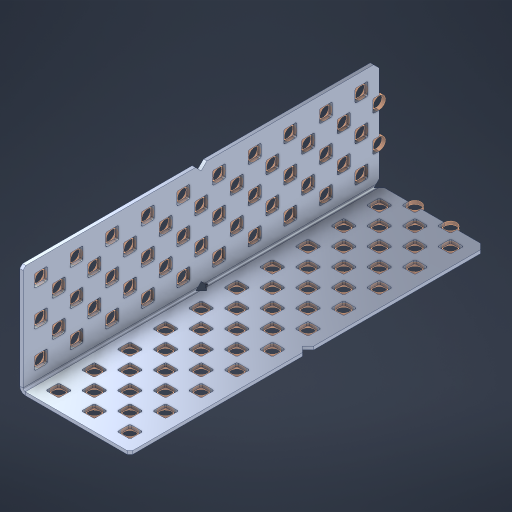
# Autodesk Inventor part: Alu C 1x2x1x35
Saved by Autodesk Inventor 2023 (Build 270158000, 158)
## iProperties
Created: 2022-07-28
Part Number: Alu C 1x2x1x35
Material: Generic
Document SubType Name: Sheet Metal
Designer: ylu12
Density: 1 g/cm^3
Sheet Metal Rule: Default
Appearance: Steel
Author: ylu12
Autodesk Inventor part; units mm, degrees
ref_plane "YZ Plane" through (0, 0, 0) normal (1, 0, 0) x (0, 1, 0)
ref_plane "XZ Plane" through (0, 0, 0) normal (0, 1, 0) x (-1, 0, 0)
sketch "Sketch1" plane through (0, 0, 0) normal (0, 1, 0) x (-1, 0, 0)
  line L0 (-19.05, 0) -> (19.05, 0)
  line L1 (19.05, 0) -> (19.05, -127)
  line L2 (19.05, -127) -> (-19.05, -127)
  line L3 (-19.05, -127) -> (-19.05, 0)
  line L4 (19.05, 0) -> (-19.05, -127) construction
  point P0 (0, 0)
  point P1 (0, 0)
  dimension "d0" = 38.1
  dimension "d1" = 127
  measures "d0" distance of L1.end L2.end
  measures "d1" distance of L0.end L1.end
extrude "Plate1" add sketch "Sketch1" along normal blind 1.1906
sketch "Sketch2" plane through (-19.05, 1.1906, 0) normal (-1, 0, 0) x (0, -1, 0)
  line L0 (0, -127) -> (0, 0)
  line L1 (0, 0) -> (-38.1, 0)
  line L2 (-38.1, 0) -> (-38.1, -127)
  line L3 (-38.1, -127) -> (0, -127)
  constraints: 6 end point, 1 horizontal, 1 perpendicular, 1 vertical
edge flange "Flanges" height 38.1 angle 90 thickness 1.1906 bend radius 0.7937 thickness toward (-1, 0, 0) relief tear relief width 1.1906 relief depth 0.5953 edges at (-19.05, 1.1906, -63.5) wall of the first edge with corners at (-19.05, 1.1906, -127) (-19.05, 1.1906, 0) (-19.05, 39.2906, 0) (-19.05, 39.2906, -127)
bend "Bend1"
corner "Corner1"
sketch "Sketch8" plane through (0, 0, 0) normal (0, -1, 0) x (1, 0, 0)
  line L0 (19.05, 0) -> (-18.2562, 0) construction
  line L1 (14.5034, -4.0386) -> (10.8966, -4.0386)
  line L2 (10.3886, -4.5466) -> (10.3886, -8.1534)
  line L3 (10.8966, -8.6614) -> (14.5034, -8.6614)
  line L4 (15.0114, -8.1534) -> (15.0114, -4.5466)
  arc A0 (15.0114, -4.5466) -> (14.5034, -4.0386) centre (14.5034, -4.5466) ccw
  arc A1 (14.5034, -8.6614) -> (15.0114, -8.1534) centre (14.5034, -8.1534) ccw
  arc A2 (10.3886, -8.1534) -> (10.8966, -8.6614) centre (10.8966, -8.1534) ccw
  arc A3 (10.8966, -4.0386) -> (10.3886, -4.5466) centre (10.8966, -4.5466) ccw
  line L5 (14.5034, -4.5466) -> (10.8966, -8.1534) construction
  line L6 (19.05, -127) -> (19.05, 0) construction
  point P0 (0, 0)
  point P1 (10.3886, -8.6614)
  point P2 (15.0114, -8.6614)
  point P3 (12.7, -6.35)
  dimension "d49" = 4.6228
  dimension "d50" = 0.508
  dimension "d52" = 6.35
  dimension "d131" = 6.35
  constraints: 10 end point, 8 point on circle, 8 tangent, 4 centre point, 4 point on line, 3 equal radius, 2 parallel, 2 perpendicular, 1 horizontal, 1 midpoint
  measures "d49" distance of point (15.011, -8.661) point (10.389, -8.661)
  measures "d50" radius of A0
  measures "d52" distance from line of L0 point (12.7, -6.35)
  measures "d131" distance from line of L6 point (12.7, -6.35)
extrude "Body Stamp" cut sketch "Sketch8" against normal blind 1.1906
sketch "Sketch9" plane through (0, 0, 0) normal (0, -1, 0) x (1, 0, 0)
  arc A0 (15.0114, -4.5466) -> (14.5034, -4.0386) centre (14.5034, -4.5466) ccw construction
  arc A1 (10.3886, -8.1534) -> (10.8966, -8.6614) centre (10.8966, -8.1534) ccw construction
  line L0 (14.5034, -4.5466) -> (10.8966, -8.1534) construction
  circle A2 centre (12.7, -6.35) radius 2.1844
  point P0 (0, 0)
  dimension "d55" = 4.3688
  constraints: 2 end point, 1 centre point, 1 midpoint
  measures "d55" diameter of A2
surface extrude "Body Circle" sketch "Sketch9" against normal up to surface (1.1906 mm away) shown yes curves A2
pattern_sketch "Body Pattern" of "Body Stamp", "Body Circle" from (12.7, 0, -6.35) copies at (0, 0, -6.35) at (-12.7, 0, -6.35) at (12.7, 0, -19.05) at (0, 0, -19.05) at (-12.7, 0, -19.05) at (12.7, 0, -31.75) at (0, 0, -31.75) at (-12.7, 0, -31.75) at (12.7, 0, -44.45) at (0, 0, -44.45) at (-12.7, 0, -44.45) at (12.7, 0, -57.15) at (0, 0, -57.15) at (-12.7, 0, -57.15) at (12.7, 0, -69.85) at (0, 0, -69.85) at (-12.7, 0, -69.85) at (12.7, 0, -82.55) at (0, 0, -82.55) at (-12.7, 0, -82.55) at (12.7, 0, -95.25) at (0, 0, -95.25) at (-12.7, 0, -95.25) at (12.7, 0, -107.95) at (0, 0, -107.95) at (-12.7, 0, -107.95) at (12.7, 0, -120.65) at (0, 0, -120.65) at (-12.7, 0, -120.65)
sketch "Sketch15" plane through (0, 0, 0) normal (0, -1, 0) x (1, 0, 0)
  line L0 (19.05, 0) -> (-18.2562, 0) construction
  line L1 (-4.5466, -10.3886) -> (-8.1534, -10.3886)
  line L2 (-8.6614, -10.8966) -> (-8.6614, -14.5034)
  line L3 (-8.1534, -15.0114) -> (-4.5466, -15.0114)
  line L4 (-4.0386, -14.5034) -> (-4.0386, -10.8966)
  arc A0 (-4.0386, -10.8966) -> (-4.5466, -10.3886) centre (-4.5466, -10.8966) ccw
  arc A1 (-4.5466, -15.0114) -> (-4.0386, -14.5034) centre (-4.5466, -14.5034) ccw
  arc A2 (-8.1534, -10.3886) -> (-8.6614, -10.8966) centre (-8.1534, -10.8966) ccw
  arc A3 (-8.6614, -14.5034) -> (-8.1534, -15.0114) centre (-8.1534, -14.5034) ccw
  line L5 (-4.5466, -10.8966) -> (-8.1534, -14.5034) construction
  line L6 (19.05, -127) -> (19.05, 0) construction
  point P0 (10.3187, 0)
  point P1 (0, 0)
  point P2 (-8.6614, -15.0114)
  point P3 (-4.0386, -15.0114)
  point P4 (-6.35, -12.7)
  dimension "d106" = 4.6228
  dimension "d107" = 0.508
  dimension "d140" = 12.7
  dimension "d141" = 25.4
  constraints: 10 end point, 8 point on circle, 8 tangent, 4 centre point, 4 point on line, 3 equal radius, 2 parallel, 2 perpendicular, 1 horizontal, 1 midpoint
  measures "d106" distance of point (-4.039, -15.011) point (-8.661, -15.011)
  measures "d107" radius of A0
  measures "d140" distance from line of L0 point (-6.35, -12.7)
  measures "d141" distance from line of L6 point (-6.35, -12.7)
extrude "Center Stamp" cut sketch "Sketch15" against normal blind 1.1906
sketch "Sketch16" plane through (0, 0, 0) normal (0, -1, 0) x (1, 0, 0)
  circle A0 centre (-6.35, -12.7) radius 2.1844
  arc A1 (-8.1534, -10.3886) -> (-8.6614, -10.8966) centre (-8.1534, -10.8966) ccw construction
  arc A2 (-4.0386, -10.8966) -> (-4.5466, -10.3886) centre (-4.5466, -10.8966) ccw construction
  line L0 (-4.5466, -10.8966) -> (-8.1534, -10.8966) construction
  arc A3 (-8.1534, -10.3886) -> (-8.6614, -10.8966) centre (-8.1534, -10.8966) ccw construction
  line L1 (-8.1534, -10.8966) -> (-6.35, -12.7) construction
  line L2 (-6.35, -12.7) -> (-4.5466, -10.8966) construction
  point P0 (0, 0)
  point P1 (10.3187, 0)
  dimension "d112" = 4.3688
  dimension "d145" = 1.8034
  constraints: 6 end point, 1 centre point, 1 horizontal, 1 perpendicular
  measures "d112" diameter of A0
  measures "d145" distance from line of L1.end L0
surface extrude "Center Circle" sketch "Sketch16" against normal up to surface (1.1906 mm away) shown yes curves A0
pattern_linear "Center Double" count 2 spacing 12.7 along (1, 0, 0) of "Center Stamp", "Center Circle"
pattern_linear "Center Pattern" count 10 spacing 12.7 along (0, 0, -1) of "Center Circle", "Center Stamp", "Center Double"
sketch "Arc Length" plane through (5.1594, 1.9844, 0) normal (0, 0, 1) x (1, 0, 0)
  line L0 (-25.4, 0) -> (-24.2094, 0) projected
  arc A0 (-25.4, 0) -> (-23.4156, -1.9844) centre (-23.4156, 0) ccw projected
  line L1 (-23.4156, -0.7938) -> (-23.4156, -1.9844) projected
  arc A1 (-24.2094, 0) -> (-23.4156, -0.7938) centre (-23.4156, 0) ccw projected
  point P0 (-5.1594, -1.9844)
  dimension "d126" = 1.2468
  dimension "d127" = 3.117
sketch "Sketch13" plane through (-20.2406, 26.5906, 317.5) normal (1, 0, 0) x (0, 0, -1)
  line L0 (378.968, 12.7) -> (381, 10.668)
  line L1 (381, 10.668) -> (383.032, 12.7)
  line L2 (378.968, 12.7) -> (383.032, 12.7)
  line L3 (381, -23.5903) -> (378.893, -25.6972)
  line L4 (378.893, -25.6972) -> (381, -27.8042)
  line L5 (381, -27.8042) -> (383.107, -25.6972)
  line L6 (383.107, -25.6972) -> (381, -23.5903)
  line L7 (381, -23.5903) -> (381, -27.8042) construction
  line L8 (381, 10.668) -> (381, -23.5903) construction
  line L9 (444.5, 12.7) -> (317.5, 12.7) projected
  line L10 (444.5, -24.6062) -> (317.5, -24.6062) construction
  line L11 (317.5, 12.7) -> (317.5, -24.6062) construction
  point P0 (444.5, -11.9062)
  point P1 (317.5, -26.5906)
  dimension "d86" = 4.2139
  dimension "d128" = 2.032
  dimension "d129" = 1.016
  dimension "d130" = 63.5
  constraints: 19 end point, 6 perpendicular, 2 vertical, 1 collinear, 1 other
  measures "d86" distance of L3.start L4.end
  measures "d128" distance from line of L2 L0.end
  measures "d130" distance between parallel lines of L11 L8
cut across bends "Notch" sketch "Sketch13" k factor 0.44
pattern_linear "Notch Pattern" count 2 spacing 63.5 along (0, 0, -1) of "Notch"
ref_plane "Diagonal Plane" through (-19.05, 1.1906, 0) normal (-0.7071068, 0.7071068, 0) x (0, 0, 1)
mirror "Everything Mirrored" about plane through (-19.05, 1.1906, 0) normal (-0.7071068, 0.7071068, 0) of "Body Stamp", "Body Circle", "Body Pattern", "Center Stamp", "Center Circle", "Center Pattern", "Notch", "Notch Pattern", "Center Double"
chamfer "End Chamfer" distance 1.016 angle 45 2 edges at (-19.6453, 39.2906, 0) (19.05, 0.5953, 0)
sketch "Body Pattern Sketch" plane through (0, 0, 0) normal (0, -1, 0) x (1, 0, 0)
  line L0 (19.05, 0) -> (-18.2562, 0) construction
  line L1 (19.05, -127) -> (19.05, 0) construction
  circle A0 centre (12.7, -6.35) radius 2.1844 construction
  point P0 (0, 0)
  point P1 (0, -6.35)
  point P2 (-12.7, -6.35)
  point P3 (12.7, -19.05)
  point P4 (0, -19.05)
  point P5 (-12.7, -19.05)
  point P6 (12.7, -31.75)
  point P7 (0, -31.75)
  point P8 (-12.7, -31.75)
  point P9 (12.7, -44.45)
  point P10 (0, -44.45)
  point P11 (-12.7, -44.45)
  point P12 (12.7, -57.15)
  point P13 (0, -57.15)
  point P14 (-12.7, -57.15)
  point P15 (12.7, -69.85)
  point P16 (0, -69.85)
  point P17 (-12.7, -69.85)
  point P18 (12.7, -82.55)
  point P19 (0, -82.55)
  point P20 (-12.7, -82.55)
  point P21 (12.7, -95.25)
  point P22 (0, -95.25)
  point P23 (-12.7, -95.25)
  point P24 (12.7, -107.95)
  point P25 (0, -107.95)
  point P26 (-12.7, -107.95)
  point P27 (12.7, -120.65)
  point P28 (0, -120.65)
  point P29 (-12.7, -120.65)
  dimension "d134" = 12.7
  dimension "d137" = 12.7
  constraints: 1 coincident, 1 horizontal, 1 vertical, 29 other
  measures "d137" distance of point (12.7, -6.35) point (0, -6.35)
equation "\"d1\" = 12.7 * Length"
equation "\"d53\" = Thickness"
equation "\"d10\" = CornerReliefSize"
equation "\"d89\" = Thickness"
equation "\"d2\" = Thickness"
equation "\"d3\" = BendReliefWidth"
equation "\"d4\" = BendReliefDepth"
equation "\"d5\" = MinimumRemnant"
equation "\"d6\" = TransitionRadius"
equation "\"d11\" = GapSize"
equation "\"d12\" = JacobiRadiusSize"
equation "\"BendRadius\" = Thickness"
equation "\"BendReliefWidth\" = Thickness"
equation "\"BendReliefDepth\" = 0.5 * Thickness"
equation "\"CornerReliefSize\" = 4 * Thickness"
equation "\"MinimumRemnant\" = 2 * Thickness"
equation "\"TransitionRadius\" = BendRadius"
equation "\"JacobiRadiusSize\" = BendRadius"
equation "\"GapSize\" = Thickness"
equation "\"Length\" = 10"
equation "\"Thickness\" = 1.190625"
body "Solid1"
body "Srf91"
body "Srf92"
body "Srf786"
body "Srf856"
body "Srf889"
body "Srf890"
body "Srf891"
body "Srf1275"
body "Srf1276"
body "Srf1278"
body "Srf1277"
body "Srf1285"
body "Srf1286"
body "Srf1287"
body "Srf1445"
body "Srf1446"
body "Srf1447"
body "Srf1448"
body "Srf1449"
body "Srf1537"
body "Srf1538"
body "Srf1539"
body "Srf1540"
body "Srf1541"
body "Srf1807"
body "Srf1959"
body "Srf2009"
body "Srf2010"
body "Srf2011"
body "Srf2012"
body "Srf2013"
body "Srf2014"
body "Srf2015"
body "Srf2016"
body "Srf2017"
body "Srf2018"
body "Srf2043"
body "Srf2044"
body "Srf2045"
body "Srf2046"
body "Srf2047"
body "Srf2048"
body "Srf2049"
body "Srf2050"
body "Srf2051"
body "Srf2076"
body "Srf2077"
body "Srf2078"
body "Srf2079"
body "Srf2080"
body "Srf2081"
body "Srf2082"
body "Srf2083"
body "Srf2084"
body "Srf2085"
body "Srf2086"
body "Srf2087"
body "Srf2088"
body "Srf2089"
body "Srf2090"
body "Srf2091"
body "Srf2092"
body "Srf2093"
body "Srf2094"
body "Srf2095"
body "Srf2096"
body "Srf2097"
body "Srf2098"
body "Srf2099"
body "Srf2100"
body "Srf2101"
body "Srf2102"
body "Srf2103"
body "Srf2179"
body "Srf2180"
body "Srf2181"
body "Srf2182"
body "Srf2183"
body "Srf2184"
body "Srf2185"
body "Srf2186"
body "Srf2187"
body "Srf2188"
body "Srf2189"
body "Srf2190"
body "Srf2191"
body "Srf2192"
body "Srf2193"
body "Srf2194"
body "Srf2195"
body "Srf2196"
body "Srf2197"
body "Srf2198"
body "Srf2199"
body "Srf2200"
body "Srf2201"
body "Srf2202"
body "Srf2203"
body "Srf2204"
body "Srf2205"
